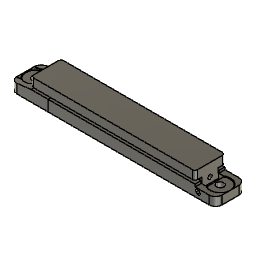
Azlestomp vstat sensor v4 (Autodesk Fusion 360 design; units mm, degrees)
Autodesk Fusion 360 part; units mm, degrees
note: some values were not read from the file. Chosen so that the rebuilt part matches the saved one: which bodies a step acts on; which face or edge a step refers to; which pieces of a blend or face edit are solid. Set by a fixed rule: which sketch regions a step uses.
sketch "Sketch1" plane through (0, 0, 0) normal (0, 0, 1) x (1, 0, 0)
  line L0 (0, 0) -> (152, 0) construction
  line L1 (152, 0) -> (152, 19.5) construction
  line L2 (152, 19.5) -> (0, 19.5) construction
  line L3 (0, 19.5) -> (0, 0) construction
  line L4 (151, 18.5) -> (1, 18.5) construction
  line L5 (1, 18.5) -> (1, 1) construction
  line L6 (1, 1) -> (151, 1) construction
  line L7 (151, 1) -> (151, 18.5) construction
  line L8 (16, 18.5) -> (136, 18.5)
  line L9 (136, 18.5) -> (136, 1)
  line L10 (136, 1) -> (16, 1)
  line L11 (16, 1) -> (16, 18.5)
  dimension "d1" = 152
  dimension "d2" = 19.5
  dimension "d3" = -1
  dimension "d4" = 17.5
  dimension "d5" = 17.5
  dimension "d6" = 120
  constraint horizontal L0
  constraint vertical L1
  constraint horizontal L2
  constraint vertical L3
  constraint coincident L0.start L3.end
  constraint horizontal L8
  constraint vertical L9
  constraint horizontal L10
  constraint vertical L11
  constraint midpoint L4 L8
  measures "d1" distance of L0.start L0.end
  measures "d2" distance of L0.start L2.end
  measures "d4" distance of L8.start L10.end
  measures "d5" distance of L4.end L5.end
  measures "d6" distance of L8.start L8.end
sketch "Sketch2" plane through (0, 0, 0) normal (0, 0, 1) x (1, 0, 0)
  circle A0 centre (22, 9.75) radius 2.15
  line L0 (16, 9.75) -> (22, 9.75) construction
  line L1 (16, 1) -> (16, 18.5) construction
  line L2 (76, 27) -> (76, 10) construction
  line L3 (151, 18.5) -> (1, 18.5) construction
  circle A1 centre (130, 9.75) radius 2.15
  dimension "d7" = 4.3
  dimension "d8" = 6
  constraint horizontal L0
  constraint midpoint L0.start L1
  constraint coincident A0.centre L0.end
  constraint vertical L2
  constraint midpoint L2 L3
  constraint symmetric A0 L2 A1
  measures "d7" diameter of A0
  measures "d8" distance of L0.start A0.centre
sketch "Sketch3" plane through (0, 0, 0) normal (0, 0, 1) x (1, 0, 0)
  line L0 (33.5, 17.25) -> (118.5, 17.25)
  line L1 (118.5, 17.25) -> (118.5, 2.25)
  line L2 (118.5, 2.25) -> (33.5, 2.25)
  line L3 (33.5, 2.25) -> (33.5, 17.25)
  line L4 (76, 18.5) -> (76, -8.2111) construction
  line L5 (151, 18.5) -> (1, 18.5) construction
  line L6 (16, 9.75) -> (141.032, 9.75) construction
  line L7 (16, 1) -> (16, 18.5) construction
  line L8 (33.5, 9.75) -> (118.5, 9.75) construction
  line L9 (76, 17.25) -> (76, 2.25) construction
  point P0 (76, 9.75)
  point P1 (76, 9.75)
  dimension "d9" = 15
  dimension "d10" = 85
  constraint horizontal L0
  constraint vertical L1
  constraint horizontal L2
  constraint vertical L3
  constraint vertical L4
  constraint midpoint L4.start L5
  constraint horizontal L6
  constraint midpoint L6.start L7
  constraint midpoint L3 L8.start
  constraint midpoint L1 L8.end
  constraint midpoint L0 L9.start
  constraint midpoint L2 L9.end
  constraint midpoint L8 P1
  constraint coincident L4 P1
  constraint coincident L6 P1
  constraint coincident P1 P0
  measures "d9" distance of L0.start L2.end
  measures "d10" distance of L0.start L0.end
extrude "Extrude1" add sketch "Sketch1" along normal blind 10 makes body 1
extrude "Extrude2" cut sketch "Sketch2" along normal blind 28 bodies 1
sketch "Sketch4" plane through (0, 0, 10) normal (0, 0, 1) x (-1, 0, 0)
  circle A0 centre (-130, -9.75) radius 2.15
  circle A1 centre (-22, -9.75) radius 2.15
  line L0 (-16, -1) -> (-136, -1)
  line L1 (-136, -1) -> (-136, -18.5)
  line L2 (-136, -18.5) -> (-16, -18.5)
  line L3 (-16, -18.5) -> (-16, -1)
  line L4 (-16, -18.5) -> (-28, -18.5)
  line L5 (-28, -18.5) -> (-28, -1)
  line L6 (-28, -1) -> (-16, -1)
  line L7 (-16, -1) -> (-16, -18.5)
  line L8 (-136, -18.5) -> (-124, -18.5)
  line L9 (-124, -18.5) -> (-124, -1)
  line L10 (-124, -1) -> (-136, -1)
  line L11 (-136, -1) -> (-136, -18.5)
  dimension "d15" = 12
  dimension "d16" = 12
  constraint horizontal L4
  constraint vertical L5
  constraint horizontal L6
  constraint vertical L7
  constraint coincident L2.end L3.start
  constraint horizontal L8
  constraint vertical L9
  constraint horizontal L10
  constraint vertical L11
  constraint coincident L1.end L2.start
  measures "d15" distance of L2.end L4.end
  measures "d16" distance of L1.end L8.end
extrude "Extrude3" cut sketch "Sketch4" against normal blind 7 contours L0 L2 L3 L4 L5 L6 L7 | L0 L1 L2 L8 L9 L10 L11 bodies 1
extrude "Extrude4" add 1 faces at (60, 6.8333, 10) along direction (0, 0, -1) blind 10 separate body on bodies 1 makes body 2
sketch "Sketch5" plane through (28, 0, 0) normal (-1, 0, 0) x (0, -1, 0)
  line L0 (-1, 10) -> (-18.5, 10)
  line L1 (-18.5, 10) -> (-18.5, 0)
  line L2 (-18.5, 0) -> (-1, 0)
  line L3 (-1, 0) -> (-1, 10)
  line L4 (-18.5, 0) -> (-18.5, 4)
  line L5 (-18.5, 4) -> (-16.5003, 5.9997)
  line L6 (-18.5, 4) -> (-15.672, 4) construction
  line L7 (-16.5003, 5.9997) -> (-16.5003, 7.5)
  line L8 (-16.5003, 7.5) -> (-18.5, 7.5)
  line L9 (-9.75, 12.0032) -> (-9.75, 10) construction
  line L10 (-18.5, 7.5) -> (-18.5, 4)
  line L11 (-1, 4) -> (-3.828, 4) construction
  line L12 (-1, 0) -> (-1, 4)
  line L13 (-1, 4) -> (-2.9997, 5.9997)
  line L14 (-1, 7.5) -> (-1, 4)
  line L15 (-2.9997, 5.9997) -> (-2.9997, 7.5)
  line L16 (-2.9997, 7.5) -> (-1, 7.5)
  dimension "d21" = 4
  dimension "d22" = 45
  dimension "d23" = 2.828
  constraint vertical L4
  constraint coincident L1.end L2.start
  constraint horizontal L6
  constraint vertical L7
  constraint coincident L1 L8.end
  constraint perpendicular L1 L8
  constraint vertical L9
  constraint midpoint L0 L9.end
  constraint symmetric L1.end L9 L2.end
  constraint symmetric L4.end L9 L11.start
  constraint symmetric L5.end L9 L13.end
  constraint symmetric L6.end L9 L11.end
  constraint symmetric L7.end L9 L15.end
  constraint symmetric L8.end L9 L14.start
  measures "d21" distance of L1.end L4.end
  measures "d22" angle of L5 L6
  measures "d23" distance of L4.end L5.end
copy_body "CopyPasteBodies1" bodies 2 makes body 3
copy_body "CopyPasteBodies2" bodies 2 makes body 4
copy_body "CopyPasteBodies3" bodies 2 makes body 5
combine "Combine1" operation cut target body 1 tool bodies 3 makes body 6 at (22.0536, 3.202, 0)
extrude "Extrude5" cut sketch "Sketch5" against normal blind 108 contours L3 L13 L14 L15 L16 | L1 L5 L7 L8 L10 bodies 4
move_face "OffsetFaces1" offset -2 6 faces at (60, 1, 1.3333) (92, 2.3331, 5.3331) (92, 2.9997, 6.4998) (60, 18.5, 2.6667) (60, 17.8334, 4.6666) (92, 16.5003, 6.4998) on bodies 4
extrude "Extrude6" cut 1 faces at (92, 12, 0) along direction (0, 0, 1) blind 2.5 on bodies 4 bodies 4
extrude "Extrude7" cut 1 faces at (28, 8.1666, 3.3904) along direction (1, 0, 0) blind 101 on bodies 4 bodies 5
move_face "OffsetFaces2" offset -0.5 9 faces at (60, 17.1668, 7.5) (60, 14.5003, 5.9475) (92, 15.8334, 3.8381) (60, 16.5, 2.7239) (60, 7.5, 2.5) (60, 3, 2.9477) (92, 3.6666, 3.8381) (60, 4.9997, 5.9475) (60, 3.6665, 7.5) on bodies 5
extrude "Extrude8" cut 2 faces at (60, 17.3334, 7) (92, 2.1666, 7) along direction (0, 0, -1) blind 0.6 on bodies 5 bodies 5
extrude "Extrude9" cut 1 faces at (60, 7.3333, 2) along direction (0, 0, -1) blind 0.6 on bodies 5 bodies 5
sketch "Sketch6" plane through (28, 0, 0) normal (-1, 0, 0) x (0, -1, 0)
  line L0 (-16.5, 2.5) -> (-3, 2.5)
  line L1 (-3, 2.5) -> (-3, 3.1716)
  line L2 (-3, 3.1716) -> (-4.9997, 5.1713)
  line L3 (-4.9997, 5.1713) -> (-4.9997, 7.5)
  line L4 (-4.9997, 7.5) -> (-1, 7.5)
  line L5 (-1, 7.5) -> (-1, 10)
  line L6 (-1, 10) -> (-18.5, 10)
  line L7 (-18.5, 10) -> (-18.5, 7.5)
  line L8 (-18.5, 7.5) -> (-14.5003, 7.5)
  line L9 (-14.5003, 7.5) -> (-14.5003, 5.1713)
  line L10 (-14.5003, 5.1713) -> (-16.5, 3.1716)
  line L11 (-16.5, 3.1716) -> (-16.5, 2.5)
  line L12 (-9.75, 2.5) -> (-9.75, 4.5) construction
  line L13 (-9.75, 4.5) -> (-14.75, 4.5) construction
  line L14 (-9.75, 4.5) -> (-4.75, 4.5) construction
  line L15 (-14.75, 4.5) -> (-4.75, 4.5)
  line L16 (-4.75, 4.5) -> (-4.75, 2.5)
  line L17 (-4.75, 2.5) -> (-14.75, 2.5)
  line L18 (-14.75, 2.5) -> (-14.75, 4.5)
  dimension "d36" = 2
  dimension "d37" = 5
  dimension "d38" = 5
  dimension "d39" = 10
  constraint midpoint L0 L12.start
  constraint perpendicular L0 L12
  constraint perpendicular L12 L13
  constraint perpendicular L12 L14
  constraint horizontal L15
  constraint vertical L16
  constraint horizontal L17
  constraint vertical L18
  measures "d36" distance of L12.start L12.end
  measures "d37" distance of L12.end L13.end
  measures "d38" distance of L12.end L14.end
  measures "d39" distance of L13.end L14.end
extrude "Extrude10" cut sketch "Sketch6" against normal blind 1 contours L0 L15 L16 L17 L18 bodies 4
sketch "Sketch7" plane through (28, 0, 0) normal (-1, 0, 0) x (0, -1, 0)
  line L0 (-4.75, 4.5) -> (-4.75, 2.5)
  line L1 (-4.75, 2.5) -> (-3, 2.5)
  line L2 (-3, 2.5) -> (-3, 3.1716)
  line L3 (-3, 3.1716) -> (-4.9997, 5.1713)
  line L4 (-4.9997, 5.1713) -> (-4.9997, 7.5)
  line L5 (-4.9997, 7.5) -> (-1, 7.5)
  line L6 (-1, 7.5) -> (-1, 10)
  line L7 (-1, 10) -> (-18.5, 10)
  line L8 (-18.5, 10) -> (-18.5, 7.5)
  line L9 (-18.5, 7.5) -> (-14.5003, 7.5)
  line L10 (-14.5003, 7.5) -> (-14.5003, 5.1713)
  line L11 (-14.5003, 5.1713) -> (-16.5, 3.1716)
  line L12 (-16.5, 3.1716) -> (-16.5, 2.5)
  line L13 (-16.5, 2.5) -> (-14.75, 2.5)
  line L14 (-14.75, 2.5) -> (-14.75, 4.5)
  line L15 (-14.75, 4.5) -> (-4.75, 4.5)
  line L16 (-9.75, 10) -> (-9.75, 4.5) construction
  circle A0 centre (-9.7456, 5.75) radius 1.25
  line L17 (-10.9955, 5.7688) -> (-11.0146, 4.5)
  line L18 (-8.4957, 5.7352) -> (-8.5103, 4.5)
  dimension "d42" = 2.5
  constraint midpoint L7 L16.start
  constraint midpoint L15 L16.end
  constraint coincident L16.end A0
  constraint coincident A0 L17.start
  constraint coincident L15 L17.end
  constraint tangent A0 L17
  constraint coincident A0 L18.start
  constraint coincident L15 L18.end
  constraint tangent A0 L18
  measures "d42" diameter of A0
extrude "Extrude11" cut sketch "Sketch7" against normal up to surface (1 mm away) contours L15 A0 L18 | L15 A0 L17 bodies 4
extrude "Extrude12" cut sketch "Sketch7" against normal blind 100 contours A0 bodies 4
fillet "Fillet1" radius 0.9 2 edges at (28.5, 11.0146, 4.5) (28.5, 8.5103, 4.5) on bodies 4
move_face "OffsetFaces3" offset -0.2 2 faces at (28.3333, 4.75, 3.8333) (28.3333, 14.75, 3.1667) on bodies 4
fillet "Fillet2" radius 0.6 2 edges at (28.5, 14.95, 4.5) (28.5, 4.55, 4.5) on bodies 4
sketch "Sketch8" plane through (0, 0, 1.4) normal (0, 0, 1) x (-1, 0, 0)
  line L0 (-124, -2.5) -> (-124, -17)
  line L1 (-124, -17) -> (-28, -17)
  line L2 (-28, -17) -> (-28, -2.5)
  line L3 (-28, -2.5) -> (-124, -2.5)
  line L4 (-124, -14.85) -> (-126, -14.85)
  line L5 (-126, -14.85) -> (-126, -4.65)
  line L6 (-126, -4.65) -> (-124, -4.65)
  line L7 (-124, -4.65) -> (-124, -14.85)
  dimension "d50" = 2
  dimension "d51" = 10.2
  constraint horizontal L4
  constraint vertical L5
  constraint horizontal L6
  constraint vertical L7
  constraint midpoint L0 L7
  measures "d50" distance of L4.start L4.end
  measures "d51" distance of L4.start L6.end
extrude "Extrude13" cut sketch "Sketch8" along normal blind 2.4 contours L0 L4 L5 L6 L7 bodies 1
extrude "Extrude14" add 2 faces at (134.7167, 9.75, 3) (21.9464, 16.298, 3) along direction (0, 0, 1) blind 2 on bodies 1 6 bodies 1 6
sketch "Sketch9" plane through (28, 0, 0) normal (-1, 0, 0) x (0, -1, 0)
  line L0 (-2.5, 3.3787) -> (-2.5, 1.4)
  line L1 (-2.5, 1.4) -> (-17, 1.4)
  line L2 (-17, 1.4) -> (-17, 3.3787)
  line L3 (-17, 3.3787) -> (-15.0003, 5.3784)
  line L4 (-15.0003, 5.3784) -> (-15.0003, 6.4)
  line L5 (-15.0003, 6.4) -> (-18.5, 6.4)
  line L6 (-18.5, 6.4) -> (-18.5, 0)
  line L7 (-18.5, 0) -> (-1, 0)
  line L8 (-1, 0) -> (-1, 6.4)
  line L9 (-1, 6.4) -> (-4.4997, 6.4)
  line L10 (-4.4997, 6.4) -> (-4.4997, 5.3784)
  line L11 (-4.4997, 5.3784) -> (-2.5, 3.3787)
  line L12 (-18.5, 0) -> (-17, 0)
  line L13 (-17, 0) -> (-17, 1.4)
  line L14 (-17, 1.4) -> (-18.5, 1.4)
  line L15 (-18.5, 1.4) -> (-18.5, 0)
  line L16 (-1, 0) -> (-2.5, 0)
  line L17 (-2.5, 0) -> (-2.5, 1.4)
  line L18 (-2.5, 1.4) -> (-1, 1.4)
  line L19 (-1, 1.4) -> (-1, 0)
  line L20 (-1, 6.4) -> (-3, 6.4)
  line L21 (-3, 6.4) -> (-3, 4.4)
  line L22 (-3, 4.4) -> (-1, 4.4)
  line L23 (-1, 4.4) -> (-1, 6.4)
  line L24 (-13.75, 0.75) -> (-5.75, 0.75)
  line L25 (-5.75, 0.75) -> (-5.75, 0)
  line L26 (-5.75, 0) -> (-13.75, 0)
  line L27 (-13.75, 0) -> (-13.75, 0.75)
  line L28 (-18.5, 0) -> (-17.5, 0)
  line L29 (-17.5, 0) -> (-17.5, 1)
  line L30 (-17.5, 1) -> (-18.5, 1)
  line L31 (-18.5, 1) -> (-18.5, 0)
  line L32 (-1, 0) -> (-2, 0)
  line L33 (-2, 0) -> (-2, 1)
  line L34 (-2, 1) -> (-1, 1)
  line L35 (-1, 1) -> (-1, 0)
  line L36 (-18.5, 6.4) -> (-16.5, 6.4)
  line L37 (-16.5, 6.4) -> (-16.5, 4.4)
  line L38 (-16.5, 4.4) -> (-18.5, 4.4)
  line L39 (-18.5, 4.4) -> (-18.5, 6.4)
  line L40 (-5.75, 0) -> (-6.7826, 1.0326)
  line L41 (-5.75, 0) -> (-4.2897, 0) construction
  line L42 (-13.75, 0) -> (-12.7247, 1.0253)
  line L43 (-13.75, 0) -> (-12.3, 0) construction
  line L44 (-18.5, 1) -> (-17.5, 0)
  line L45 (-2, 0) -> (-1, 1)
  line L46 (-3, 5.4) -> (-2, 4.4)
  line L47 (-17.5, 4.4) -> (-16.5, 5.4)
  line L48 (-18.5, 1.4) -> (-17, 0)
  line L49 (-2.5, 0) -> (-1, 1.4)
  dimension "d56" = 2
  dimension "d57" = 2
  dimension "d58" = 8
  dimension "d59" = 0.75
  dimension "d60" = 1
  dimension "d61" = 1
  dimension "d62" = 1
  dimension "d63" = 1
  dimension "d64" = 2
  dimension "d65" = 2
  dimension "d68" = 135
  dimension "d69" = 45
  constraint horizontal L12
  constraint vertical L13
  constraint horizontal L14
  constraint vertical L15
  constraint coincident L1.end L2.start
  constraint coincident L6.end L7.start
  constraint horizontal L16
  constraint vertical L17
  constraint horizontal L18
  constraint vertical L19
  constraint coincident L0.end L1.start
  constraint coincident L7.end L8.start
  constraint horizontal L20
  constraint vertical L21
  constraint horizontal L22
  constraint vertical L23
  constraint coincident L8.end L9.start
  constraint horizontal L24
  constraint vertical L25
  constraint horizontal L26
  constraint vertical L27
  constraint midpoint L7 L26
  constraint horizontal L28
  constraint vertical L29
  constraint horizontal L30
  constraint vertical L31
  constraint horizontal L32
  constraint vertical L33
  constraint horizontal L34
  constraint vertical L35
  constraint horizontal L36
  constraint vertical L37
  constraint horizontal L38
  constraint vertical L39
  constraint coincident L5.end L6.start
  constraint horizontal L41
  constraint horizontal L43
  constraint midpoint L21 L46.start
  constraint midpoint L22 L46.end
  constraint midpoint L38 L47.start
  constraint midpoint L37 L47.end
  measures "d56" distance of L8.end L20.end
  measures "d57" distance of L8.end L22.end
  measures "d58" distance of L24.start L24.end
  measures "d59" distance of L24.start L26.end
  measures "d60" distance of L6.end L28.end
  measures "d61" distance of L6.end L30.end
  measures "d62" distance of L7.end L32.end
  measures "d63" distance of L7.end L34.end
  measures "d64" distance of L5.end L36.end
  measures "d65" distance of L5.end L38.end
  measures "d68" angle of L40 L41
  measures "d69" angle of L42 L43
extrude "Extrude15" add sketch "Sketch9" against normal blind 10 separate body contours L7 L16 L33 L49 | L8 L19 L34 L49 | L7 L12 L29 L48 | L6 L15 L30 L48 | L7 L24 L26 L40 L42 | L7 L8 L16 L19 L32 L35 L45 | L33 L34 L45 L49 | L8 L9 L20 L21 L22 L23 L46 | L29 L30 L44 L48 | L6 L7 L12 L15 L28 L31 L44 | L5 L6 L36 L37 L38 L39 L47 makes body 7 at (31.3333, 11.0833, 0) makes body 8 at (31.3333, 18, 0.9333) makes body 9 at (31.3333, 2, 0.4667) makes body 10 at (34.6667, 18.5, 5.7333) makes body 11 at (34.6667, 1.6667, 6.4)
copy_body "CopyPasteBodies4" bodies 7 10 9 8 11 makes body 12 makes body 13 makes body 14 makes body 15 makes body 16
move_body "Move1" bodies 12 13 14 15 16 to x (1, 0, 0) y (0, 1, 0) z (0, 0, 1) at (86, 0, 0)
sketch "circle cutout" plane through (0, 1, 0) normal (0, -1, 0) x (1, 0, 0)
  line L0 (124, 5) -> (124, 0)
  line L1 (124, 0) -> (136, 0)
  line L2 (136, 0) -> (136, 5)
  line L3 (136, 5) -> (124, 5)
  circle A0 centre (125.3681, 3.5411) radius 1
  circle A1 centre (126.0752, 2.834) radius 1
  line L4 (125.3681, 3.5411) -> (126.0752, 2.834)
  line L5 (125.3681, 3.5411) -> (126.3681, 3.5411) construction
  line L6 (126.0752, 2.834) -> (125.3681, 3.5411)
  line L7 (125.3681, 3.5411) -> (126.0752, 4.2482)
  line L8 (126.0752, 4.2482) -> (126.7823, 3.5411)
  line L9 (126.7823, 3.5411) -> (126.0752, 2.834)
  line L10 (126.0752, 2.834) -> (125.3681, 3.5411)
  line L11 (125.3681, 3.5411) -> (124.661, 2.834)
  line L12 (124.661, 2.834) -> (125.3681, 2.1269)
  line L13 (125.3681, 2.1269) -> (126.0752, 2.834)
  dimension "d94" = 2
  dimension "d97" = 2
  dimension "d98" = 1
  dimension "d99" = 45
  constraint horizontal L5
  constraint coincident A0.centre L4.start
  constraint coincident A1.centre L4.end
  constraint perpendicular L6 L7
  constraint parallel L6 L8
  constraint parallel L7 L9
  constraint parallel L4 L6
  constraint perpendicular L10 L11
  constraint parallel L10 L12
  constraint parallel L11 L13
  constraint perpendicular L7 L10
  measures "d94" diameter of A0
  measures "d97" diameter of A1
  measures "d98" distance of A0.centre A1.centre
  measures "d99" angle of L4 L5
extrude "Extrude16" cut sketch "circle cutout" against normal blind 4.5 contours A0 L7 L11 | A0 A1 L8 | A0 A1 L7 | A0 A1 L11 | A0 A1 L12 | A0 A1 L9 | A0 A1 L4 L6 L10 | A0 A1 L4 L6 L10 | A1 L9 L13 | A0 A1 L13 bodies 1
delete_body "RemoveBody1" bodies 16
delete_body "RemoveBody2" bodies 14
delete_body "RemoveBody3" bodies 12
delete_body "RemoveBody4" bodies 13
delete_body "RemoveBody5" bodies 15
sketch "Sketch11" plane through (0, 18.5, 0) normal (0, 1, 0) x (-1, 0, 0)
  line L0 (-28, 5) -> (-28, 0)
  line L1 (-28, 0) -> (-16, 0)
  line L2 (-16, 0) -> (-16, 5)
  line L3 (-16, 5) -> (-28, 5)
  line L4 (-28, 6.4) -> (-16, 5)
  line L5 (-28, 6.4) -> (-28, 5)
  constraint coincident L2.end L3.start
  constraint coincident L0.start L3.end
extrude "Extrude17" add sketch "Sketch11" against normal blind 3.5 separate body contours L3 L4 L5 makes body 17
extrude "Extrude18" add sketch "Sketch11" along normal blind -14 and the other way blind 17.5 separate body contours L3 L4 L5 makes body 18
combine "Combine2" operation add target body 6 tool bodies 8 17 18 11 7 10 9
copy_body "CopyPasteBodies5" bodies 6 makes body 19
combine "Combine3" operation cut target body 5 tool bodies 19
combine "Combine4" operation add target body 5 tool bodies 1
sketch "Sketch12" plane through (0, 0, 5) normal (0, 0, 1) x (-1, 0, 0)
  line L0 (-16, -4.5) -> (-28, -4.5)
  line L1 (-28, -4.5) -> (-28, -15)
  line L2 (-28, -15) -> (-16, -15)
  line L3 (-16, -15) -> (-16, -4.5)
  circle A0 centre (-22, -9.75) radius 2.15
  circle A1 centre (-22, -9.75) radius 5.75
  dimension "d78" = 11.5
  constraint concentric A0 A1
  measures "d78" diameter of A1
sketch "Sketch13" plane through (0, 0, 5) normal (0, 0, 1) x (-1, 0, 0)
  line L0 (-124, -14.85) -> (-126, -14.85)
  line L1 (-126, -14.85) -> (-126, -4.65)
  line L2 (-126, -4.65) -> (-124, -4.65)
  line L3 (-124, -4.65) -> (-124, -4.1213)
  line L4 (-124, -4.1213) -> (-124, -1)
  line L5 (-124, -1) -> (-136, -1)
  line L6 (-136, -1) -> (-136, -18.5)
  line L7 (-136, -18.5) -> (-124, -18.5)
  line L8 (-124, -18.5) -> (-124, -15.3787)
  line L9 (-124, -15.3787) -> (-124, -14.85)
  circle A0 centre (-130, -9.75) radius 2.15
  circle A1 centre (-130, -9.75) radius 5.75
  dimension "d79" = 11.5
  constraint concentric A0 A1
  measures "d79" diameter of A1
extrude "Extrude19" cut sketch "Sketch12" sketch "Sketch13" along normal blind 8 and the other way blind 0.3 contours L0 L2 A1 | L0 A1 | L2 A1 of sketch 2 contours L1 A1 | L1 A1 bodies 5 6
fillet "Fillet3" radius 0.35 5 edges at (135.75, 9.75, 5) (27.75, 9.75, 5) (16.25, 9.75, 5) (22, 15.5, 5.7) (22, 4, 5.7) on bodies 5 6
fillet "Fillet4" radius 3.75 4 edges at (136, 1, 2.5) (136, 18.5, 2.5) (16, 1, 2.5) (16, 18.5, 2.5) on bodies 5 6
extrude "Extrude20" add 2 faces at (31.3333, 17.8333, 4.4) (31.3333, 1.6667, 4.4) along direction (0, 0, -1) blind 4 on bodies 6 bodies 6
extrude "Extrude21" cut 2 faces at (31.3333, 17.8333, 4.4) (31.3333, 1.6667, 4.4) along direction (0, 0, -1) blind 5 on bodies 5 bodies 5
move_face "OffsetFaces4" offset 0.2 6 faces at (31.3333, 17.5, 3.0889) (34.6667, 17.1667, 4.7333) (34.6667, 17.1667, 0.1556) (31.3333, 2.3333, 0.1556) (34.6667, 2, 1.7778) (34.6667, 2.6667, 5.0667) on bodies 5
move_face "OffsetFaces5" offset -0.2 6 faces at (34.6667, 2, 1.7778) (34.6667, 2.6667, 5.0667) (31.3333, 2.3333, 0.1556) (31.3333, 17.5, 3.0889) (34.6667, 17.1667, 4.7333) (34.6667, 17.1667, 0.1556) on bodies 6
move_face "OffsetFaces6" offset 0.1 2 faces at (95.3333, 17, 2.7191) (95.3333, 2.5, 2.7191) on bodies 5
move_face "OffsetFaces7" offset -0.2 1 faces at (34.6667, 10.8333, 0.75) on bodies 5
extrude "Extrude22" cut 1 faces at (126, 11.4119, 2.6456) along direction (1, 0, 0) blind 1 on bodies 5 bodies 5
extrude "Extrude23" add 1 faces at (60, 6.8333, 10) along direction (0, 0, 1) blind 3 on bodies 4 bodies 4
extrude "Extrude24" cut 2 faces at (60, 3.6665, 7.5) (92, 17.1668, 7.5) along direction (0, 0, 1) blind 0.5 on bodies 4 bodies 4
fillet "Fillet5" radius 1.5 4 edges at (28, 18.5, 10.5) (28, 1, 10.5) (124, 1, 10.5) (124, 18.5, 10.5) on bodies 4
hidden bodies 2
equation "d23 = 1.414 mm * 2"
named bodies: "wire boi", "Master extrude", "top", "bottom", "spike boi", "spike boi (1)"
